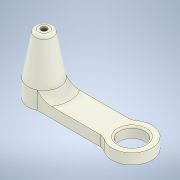
# Autodesk Inventor part: LinkA
Saved by Autodesk Inventor 2022 (Build 260153000, 153)
## iProperties
Created: 2021-11-22
Part Number: LinkA
Material: Plástico ABS
Document SubType Name: Modeling
Designer: JK
Density: 1.06 g/cm^3
Appearance: Suave - Marfil
Author: JK
Autodesk Inventor part; units mm, degrees
ref_plane "YZ Plane" through (0, 0, 0) normal (1, 0, 0) x (0, 1, 0)
ref_plane "XZ Plane" through (0, 0, 0) normal (0, 1, 0) x (-1, 0, 0)
ref_plane "XY Plane" through (0, 0, 0) normal (0, 0, 1) x (1, 0, 0)
sketch "Boceto1" plane through (0, 0, 0) normal (0, 1, 0) x (-1, 0, 0)
  circle A0 centre (0, 0) radius 4
  circle A1 centre (0, 0) radius 1.65
  line L0 (0, 4) -> (-25, 4)
  line L1 (-25, 4) -> (-25, -4)
  line L2 (-25, -4) -> (0, -4)
  line L3 (0, -4) -> (0, 4)
  circle A2 centre (-25, 0) radius 4
  circle A3 centre (-25, 0) radius 1.65
  line L4 (-1.27, 1.0534) -> (-1.27, -1.0534)
  point P0 (-25, 4)
  point P1 (0, -4)
  dimension "d1" = 8
  dimension "d0" = 3.3
  dimension "d2" = 25
  dimension "d3" = 3.3
  dimension "d4" = 1.27
  constraints: 10 end point, 3 coincident, 3 horizontal, 2 centre point, 2 parallel, 2 point on circle, 1 midpoint, 1 perpendicular, 1 vertical, 6 other
  measures "d0" diameter of A1
  measures "d2" distance from line of point (0, 0) L1
  measures "d3" diameter of A3
  measures "d4" distance from line of point (0, 0) L4
extrude "Extrusión1" add sketch "Boceto1" along normal blind 5 contours A0 L3 A1 | L3 A1 A0 | A0 L2 A2 L0 | A2 L1 A3 | L1 A3 A2 | L4 A1
sketch "Boceto5" plane through (0, 5, 0) normal (0, 1, 0) x (1, 0, 0)
  circle A0 centre (0, 0) radius 4.5
  dimension "d12" = 9
  constraints: 1 centre point, 1 coincident
  measures "d12" diameter of A0
extrude "Extrusión4" add sketch "Boceto5" along normal blind 12 draft -10
sketch "Boceto8" plane through (0, 17, 0) normal (0, 1, 0) x (1, 0, 0)
  circle A0 centre (0, 0) radius 0.85
  dimension "d21" = 1.7
  constraints: 1 centre point, 1 coincident
  measures "d21" diameter of A0
extrude "Extrusión5" cut sketch "Boceto8" against normal blind 6.5
sketch "Boceto9" plane through (0, 0, 0) normal (0, -1, 0) x (1, 0, 0)
  arc A0 (2.0616, 4) -> (2.0616, -4) centre (0, 0) ccw projected
  arc A1 (2.0616, -4) -> (2.0616, 4) centre (0, 0) ccw projected
  line L0 (25, -4) -> (0, -4) projected
  arc A2 (25, -4) -> (25, 4) centre (25, 0) ccw projected
  line L1 (0, 4) -> (25, 4) projected
  arc A3 (0, 4) -> (0, -4) centre (0, 0) ccw projected
  arc A4 (1.27, 1.0534) -> (1.27, -1.0534) centre (0, 0) ccw projected
  line L2 (1.27, -1.0534) -> (1.27, 1.0534) projected
  circle A5 centre (25, 0) radius 1.65 projected
  point P0 (2.0616, -4)
extrude "Extrusión6" add sketch "Boceto9" against normal up to surface (5 mm away) contours L1 A3 L0 A0
sketch "Boceto11" plane through (0, 10.5, 0) normal (0, 1, 0) x (1, 0, 0)
  circle A0 centre (0, 0) radius 0.85 projected
extrude "Extrusión7" cut sketch "Boceto11" against normal blind 1.5
sketch "Boceto12" plane through (0, 5, 0) normal (0, 1, 0) x (1, 0, 0)
  arc A0 (2.0616, -4) -> (2.0616, 4) centre (0, 0) ccw projected
  line L0 (2.0616, -4) -> (25, -4) projected
  arc A1 (25, -4) -> (25, 4) centre (25, 0) ccw projected
  line L1 (25, 4) -> (2.0616, 4) projected
  circle A2 centre (25, 0) radius 1.65 projected
extrude "Extrusión8" cut sketch "Boceto12" against normal blind 2
sketch "Boceto14" plane through (0, 3, 0) normal (0, 1, 0) x (1, 0, 0)
  circle A0 centre (25, 0) radius 1.65 projected
  circle A1 centre (25, 0) radius 3.65
  circle A2 centre (25, 0) radius 5.65
  point P0 (0, 0)
  dimension "d36" = 7.3
  dimension "d37" = 2
  constraints: 2 centre point, 2 coincident
  measures "d36" diameter of A1
  measures "d37" radial gap between concentric circles of A2 A1
extrude "Extrusión9" add sketch "Boceto14" against normal up to surface (3 mm away) contours A2
sketch "Boceto15" plane through (0, 3, 0) normal (0, 1, 0) x (1, 0, 0)
  circle A0 centre (25, 0) radius 3.6
  point P0 (0, 0)
  dimension "d43" = 7.2
  constraints: 1 centre point, 1 coincident
  measures "d43" diameter of A0
extrude "Extrusión10" cut sketch "Boceto15" against normal through all
fillet "Empalme1" radius 3 3 edges at (21.0097, 1.5, 4) (21.0097, 1.5, -4) (4.5, 3, 0)
sketch "Boceto17" plane through (0, 9, 0) normal (0, 1, 0) x (1, 0, 0)
  circle A0 centre (0, 0) radius 0.85 projected
  line L0 (0.85, 0) -> (-0.85, 0)
  circle A1 centre (0, 0) radius 0.85 projected
  constraints: 2 end point, 2 point on circle, 1 horizontal
extrude "Extrusión12" add sketch "Boceto17" along normal blind 1.5 contours L0 A0 picked at (0.2121, 0.1879)
fillet "Empalme2" radius 1 1 edges at (-2.3841, 17, 0)
fillet "Empalme3" radius 0.5 1 edges at (21.4, 3, 0)
sketch "Boceto18" plane through (0, 5, 0) normal (0, -1, 0) x (1, 0, 0)
  arc A0 (0.85, 0) -> (-0.85, 0) centre (0, 0) ccw projected
  line L0 (1.27, -1.0534) -> (1.27, 1.0534) projected
  arc A1 (1.27, 1.0534) -> (1.27, -1.0534) centre (0, 0) ccw projected
extrude "Extrusión13" cut sketch "Boceto18" against normal blind 3
sketch "Boceto16" plane through (0, 0, 0) normal (0, -1, 0) x (1, 0, 0)
  circle A0 centre (25, 0) radius 3.6 projected
  circle A1 centre (25, 0) radius 3
  point P0 (0, 0)
  dimension "d44" = 6
  dimension "d35" = 17.0679
  constraints: 1 centre point, 1 coincident
  measures "d35" diameter of A1
sketch "Boceto6" plane through (0, 17, 0) normal (0, 1, 0) x (1, 0, 0)
  circle A0 centre (0, 0) radius 4.5
  dimension "d15" = 9
  constraints: 1 centre point, 1 coincident
  measures "d15" diameter of A0
sketch "Boceto7" plane through (0, 5, 0) normal (0, 1, 0) x (1, 0, 0)
  arc A0 (1.27, 1.0534) -> (1.27, -1.0534) centre (0, 0) ccw projected
  circle A1 centre (0, 0) radius 4
  dimension "d16" = 8
  constraints: 1 centre point, 1 coincident
  measures "d16" diameter of A1
sketch "Boceto2" plane through (0, 5, 0) normal (0, 1, 0) x (1, 0, 0)
  line L0 (40, 3) -> (0, 3) projected
  arc A0 (0, 3) -> (0, -3) centre (0, 0) ccw projected
  line L1 (0, -3) -> (40, -3) projected
  arc A1 (40, -3) -> (40, 3) centre (40, 0) ccw projected
  arc A2 (1.27, 1.0534) -> (1.27, -1.0534) centre (0, 0) ccw projected
  line L2 (1.27, 1.0534) -> (1.27, -1.0534) projected
  circle A3 centre (40, 0) radius 1.65 projected
sketch "Boceto4" plane through (0, 6.2, 0) normal (0, 1, 0) x (1, 0, 0)
  arc A0 (1.27, 1.0534) -> (1.27, -1.0534) centre (0, 0) ccw projected
  circle A1 centre (0, 0) radius 5
  dimension "d9" = 10
  constraints: 1 centre point, 1 coincident
  measures "d9" diameter of A1
